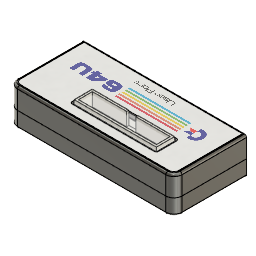
C64U UserPort Case (Autodesk Fusion 360 design; units mm, degrees)
part number: 2026-07-06-14-41-17-070
part number: 2026-07-06-14-41-58-106
part number: 2026-07-06-16-35-42-288
part number: 2026-07-06-17-32-42-446
part number: 2026-07-06-18-13-47-338
Autodesk Fusion 360 part; units mm, degrees
note: some values were not read from the file. Chosen so that the rebuilt part matches the saved one: which bodies a step acts on; the layout of a text. Set by a fixed rule: which sketch regions a step uses.
sketch "Sketch1" plane through (0, 0, 0) normal (0, 0, 1) x (1, 0, 0) in component "PCB"
  line L0 (49.1, 33.3) -> (2, 33.3)
  line L1 (0, 31.3) -> (0, 2)
  arc A0 (2, 33.3) -> (0, 31.3) centre (2, 31.3) ccw
  arc A1 (51.1, 31.3) -> (49.1, 33.3) centre (49.1, 31.3) ccw
  arc A2 (0, 2) -> (2, 0) centre (2, 2) ccw
  arc A3 (49.1, 0) -> (51.1, 2) centre (49.1, 2) ccw
  arc A4 (7.5, 0) -> (4.5, 0) centre (6, 0) ccw
  line L2 (2, 0) -> (4.5, 0)
  line L3 (7.5, 0) -> (49.1, 0)
  arc A5 (51.1, 20) -> (51.1, 17) centre (51.1, 18.5) ccw
  line L4 (51.1, 2) -> (51.1, 17)
  line L5 (51.1, 20) -> (51.1, 31.3)
  line L6 (9.9, 4.5) -> (50.4, 4.5)
  line L7 (50.4, 4.5) -> (50.4, 13.5)
  line L8 (50.4, 13.5) -> (9.9, 13.5)
  line L9 (9.9, 13.5) -> (9.9, 4.5)
  line L10 (11, 5.6) -> (49.3, 5.6)
  line L11 (49.3, 5.6) -> (49.3, 12.4)
  line L12 (49.3, 12.4) -> (11, 12.4)
  line L13 (11, 12.4) -> (11, 5.6)
  line L14 (30.15, 13.5) -> (30.15, 4.5) construction
  line L15 (32.4, 12.4) -> (32.4, 13.5)
  line L16 (27.9, 13.5) -> (27.9, 12.4)
  line L17 (14.55, 21.8) -> (36.55, 21.8)
  line L18 (36.55, 21.8) -> (36.55, 19.8)
  line L19 (36.55, 19.8) -> (14.55, 19.8)
  line L20 (14.55, 19.8) -> (14.55, 21.8)
  line L21 (25.55, 33.3) -> (25.55, 0) construction
  dimension "d3" = 2
  dimension "d4" = 2
  dimension "d5" = 2
  dimension "d6" = 2
  dimension "d7" = 33.3
  dimension "d8" = 51.1
  dimension "d9" = 3
  dimension "d10" = 6
  dimension "d11" = 3
  dimension "d12" = 18.5
  dimension "d13" = 40.5
  dimension "d14" = 9
  dimension "d15" = 0.7
  dimension "d16" = 4.5
  dimension "d17" = -1.1
  dimension "d18" = 4.5
  dimension "d19" = 22
  dimension "d20" = 2
  dimension "d21" = 11.5
  constraint horizontal L2
  constraint vertical L4
  constraint horizontal L0
  constraint vertical L1
  constraint tangent L0 A0
  constraint tangent L1 A0
  constraint tangent A1 L5
  constraint tangent L0 A1
  constraint tangent A2 L2
  constraint tangent L1 A2
  constraint tangent A3 L3
  constraint tangent A3 L4
  constraint coincident A4.centre L2
  constraint collinear L2 L3
  constraint coincident A5.centre L4
  constraint collinear L4 L5
  constraint horizontal L6
  constraint vertical L7
  constraint horizontal L8
  constraint vertical L9
  constraint midpoint L8 L14.start
  constraint midpoint L6 L14.end
  constraint coincident L12 L15.start
  constraint coincident L8 L15.end
  constraint perpendicular L8 L15
  constraint coincident L8 L16.start
  constraint coincident L12 L16.end
  constraint perpendicular L12 L16
  constraint symmetric L14 L15 L16
  constraint horizontal L17
  constraint vertical L18
  constraint horizontal L19
  constraint vertical L20
  constraint midpoint L0 L21.start
  constraint coincident L3 L21.end
  constraint perpendicular L3 L21
  constraint symmetric L18 L20 L21
  measures "d3" radius of A0
  measures "d4" radius of A1
  measures "d5" radius of A2
  measures "d6" radius of A3
  measures "d7" distance of L0 L2
  measures "d8" distance of L1 L4
  measures "d9" diameter of A4
  measures "d10" distance of L1 A4.centre
  measures "d11" diameter of A5
  measures "d12" distance of L3 A5.centre
  measures "d13" distance of L7 L9
  measures "d14" distance of L6.end L7.end
  measures "d15" distance of L4 L7
  measures "d16" distance of L3 L6
  measures "d18" distance of L15 L16
  measures "d19" distance of L18 L20
  measures "d20" distance of L17 L19
  measures "d21" distance of L0 L17
extrude "Extrude1" add sketch "Sketch1" against normal blind 1.6 contours L0 L1 A0 A1 A2 A3 A4 L2 L3 A5 L4 L5 | L6 L7 L8 L9 L10 L11 L12 L13 L15 L16 | L8 L12 L15 L16 | L10 L11 L12 L13 | L17 L18 L19 L20 makes body 1 in component "PCB"
extrude "Extrude2" add sketch "Sketch1" along normal blind 9.5 contours L6 L7 L8 L9 L10 L11 L12 L13 L15 L16 bodies 1 in component "PCB"
extrude "Extrude3" add sketch "Sketch1" along normal blind 3 contours L8 L12 L15 L16 | L10 L11 L12 L13 bodies 1 in component "PCB"
ref_plane "WorkPlane1" through (25.55, 16.65, -7.9) normal (0, 0, 1) x (1, 0, 0) in component "bottom_shell"
sketch "Sketch1 (2)" plane through (0, 0, -7.9) normal (0, 0, 1) x (1, 0, 0) in component "bottom_shell"
  line L0 (49.1, 33.3) -> (2, 33.3) construction
  arc A0 (2, 33.3) -> (0, 31.3) centre (2, 31.3) ccw construction
  line L1 (0, 31.3) -> (0, 2) construction
  arc A1 (0, 2) -> (2, 0) centre (2, 2) ccw construction
  line L2 (2, 0) -> (4.5, 0) construction
  arc A2 (7.5, 0) -> (4.5, 0) centre (6, 0) ccw construction
  line L3 (7.5, 0) -> (49.1, 0) construction
  arc A3 (49.1, 0) -> (51.1, 2) centre (49.1, 2) ccw construction
  line L4 (51.1, 2) -> (51.1, 17) construction
  arc A4 (51.1, 20) -> (51.1, 17) centre (51.1, 18.5) ccw construction
  line L5 (51.1, 20) -> (51.1, 31.3) construction
  arc A5 (51.1, 31.3) -> (49.1, 33.3) centre (49.1, 31.3) ccw construction
  line L6 (25.55, 33.3) -> (25.55, 0) construction
  line L7 (50.4, 13.5) -> (9.9, 13.5) construction
  line L8 (9.9, 13.5) -> (9.9, 4.5) construction
  line L9 (9.9, 4.5) -> (50.4, 4.5) construction
  line L10 (50.4, 4.5) -> (50.4, 13.5) construction
  line L11 (14.55, 21.8) -> (36.55, 21.8) construction
  line L12 (36.55, 19.8) -> (14.55, 19.8) construction
  circle A6 centre (-4.5, 17.8) radius 4
  circle A7 centre (-4.5, 3.5) radius 4
  line L13 (-14.95, 33.3) -> (66.05, 33.3)
  line L14 (66.05, 33.3) -> (66.05, 1.5)
  line L15 (62.05, -2.5) -> (-10.95, -2.5)
  line L16 (-14.95, 1.5) -> (-14.95, 33.3)
  line L17 (-12.95, 33.3) -> (-12.95, 1.5)
  line L18 (-10.95, -0.5) -> (62.05, -0.5)
  line L19 (64.05, 1.5) -> (64.05, 33.3)
  arc A8 (-12.95, 1.5) -> (-10.95, -0.5) centre (-10.95, 1.5) ccw
  arc A9 (62.05, -0.5) -> (64.05, 1.5) centre (62.05, 1.5) ccw
  arc A10 (-14.95, 1.5) -> (-10.95, -2.5) centre (-10.95, 1.5) ccw
  arc A11 (62.05, -2.5) -> (66.05, 1.5) centre (62.05, 1.5) ccw
  line L20 (4.8, 0) -> (4.8, -0.5)
  line L21 (7.2, 0) -> (7.2, -0.5)
  arc A12 (7.2, -0.0006) -> (4.8, 0) centre (6, 0) ccw
  line L22 (6, 0) -> (6, -0.5) construction
  line L23 (3.5, -0.5) -> (8.5, -0.5)
  line L24 (8.5, -0.5) -> (8.5, 2.5)
  line L25 (8.5, 2.5) -> (3.5, 2.5)
  line L26 (3.5, 2.5) -> (3.5, -0.5)
  line L27 (-12.95, 7.5) -> (2.5, 7.5)
  line L28 (2.5, 7.5) -> (2.5, -0.5)
  line L29 (-0.3, 7.5) -> (-0.3, -0.5)
  line L30 (-12.95, 21.8) -> (2.5, 21.8)
  line L31 (2.5, 21.8) -> (2.5, 13.8)
  line L32 (2.5, 13.8) -> (-12.95, 13.8)
  line L33 (-0.3, 21.8) -> (-0.3, 13.8)
  circle A13 centre (-4.5, 17.8) radius 3
  circle A14 centre (-4.5, 3.5) radius 3
  line L34 (64.05, 21.8) -> (48.6, 21.8)
  circle A15 centre (55.6, 17.8) radius 4
  circle A16 centre (55.6, 17.8) radius 3
  line L35 (48.6, 13.8) -> (64.05, 13.8)
  line L36 (51.4, 21.8) -> (51.4, 13.8)
  line L37 (48.6, 21.8) -> (48.6, 13.8)
  line L38 (64.05, 7.5) -> (48.6, 7.5)
  circle A17 centre (55.6, 3.5) radius 4
  circle A18 centre (55.6, 3.5) radius 3
  line L39 (51.4, 7.5) -> (51.4, -0.5)
  line L40 (48.6, 7.5) -> (48.6, -0.5)
  circle A19 centre (-4.5, 17.8) radius 1.75
  circle A20 centre (-4.5, 3.5) radius 1.75
  circle A21 centre (55.6, 17.8) radius 1.75
  circle A22 centre (55.6, 3.5) radius 1.75
  line L41 (2.5, 21.8) -> (48.6, 21.8)
  line L42 (2.5, 19.8) -> (48.6, 19.8)
  line L43 (64.85, 32.1) -> (64.85, 1.5)
  arc A23 (62.05, -1.3) -> (64.85, 1.5) centre (62.05, 1.5) ccw
  line L44 (62.05, -1.3) -> (-10.95, -1.3)
  arc A24 (-13.75, 1.5) -> (-10.95, -1.3) centre (-10.95, 1.5) ccw
  line L45 (-13.75, 1.5) -> (-13.75, 32.1)
  line L46 (-13.75, 32.1) -> (-13.75, 33.3)
  line L47 (64.85, 32.1) -> (64.85, 33.3)
  line L48 (51.1, 20) -> (51.1, 17) construction
  line L49 (51.4, 19.7) -> (51.1, 19.7)
  arc A25 (51.1, 19.7) -> (51.1, 17.3) centre (51.1, 18.5) ccw
  line L50 (51.1, 18.5) -> (50.5645, 18.5) construction
  line L51 (51.4, 17.3) -> (51.1, 17.3)
  point P0 (4.5, 0)
  dimension "d34" = 8
  dimension "d35" = 8
  dimension "d37" = 4.5
  dimension "d39" = 4.5
  dimension "d41" = 4
  dimension "d42" = 2.5
  dimension "d43" = 81
  dimension "d44" = 2
  dimension "d45" = 2
  dimension "d46" = 2
  dimension "d47" = 2
  dimension "d48" = 4
  dimension "d49" = 4
  dimension "d50" = 0.3
  dimension "d51" = 0.3
  dimension "d52" = 5
  dimension "d53" = 3
  dimension "d54" = 2.5
  dimension "d55" = 0.3
  dimension "d56" = 6
  dimension "d57" = 6
  dimension "d58" = 3.5
  dimension "d59" = 3.5
  dimension "d60" = 2
  dimension "d61" = 1.2
  dimension "d63" = 0.3
  constraint horizontal L13
  constraint vertical L14
  constraint horizontal L15
  constraint vertical L16
  constraint collinear L0 L13
  constraint symmetric L6 L14 L16
  constraint coincident L13 L17.start
  constraint perpendicular L13 L17
  constraint perpendicular L14 L18
  constraint coincident L13 L19.end
  constraint perpendicular L13 L19
  constraint symmetric L6 L17 L19
  constraint tangent L17 A8
  constraint tangent L18 A8
  constraint tangent L18 A9
  constraint tangent L19 A9
  constraint tangent L15 A10
  constraint tangent L16 A10
  constraint tangent L14 A11
  constraint tangent L15 A11
  constraint concentric A2 A12
  constraint coincident L18 L20.end
  constraint perpendicular L18 L20
  constraint coincident L21.start A12
  constraint coincident L18 L21.end
  constraint perpendicular L18 L21
  constraint coincident L21 A12.start
  constraint coincident A2.centre A12.centre
  constraint coincident L18 L22.end
  constraint perpendicular L18 L22
  constraint horizontal L23
  constraint vertical L24
  constraint horizontal L25
  constraint vertical L26
  constraint coincident L18 L23.start
  constraint symmetric L22 L24 L26
  constraint coincident L17 L27.start
  constraint perpendicular L1 L27
  constraint coincident L18 L28.end
  constraint perpendicular L18 L28
  constraint tangent A7 L27
  constraint coincident L27 L29.start
  constraint coincident L18 L29.end
  constraint perpendicular L18 L29
  constraint coincident L17 L30.start
  constraint perpendicular L1 L30
  constraint perpendicular L30 L31
  constraint coincident L17 L32.end
  constraint perpendicular L17 L32
  constraint collinear L28 L31
  constraint tangent A6 L30
  constraint tangent A6 L32
  constraint coincident L30 L33.start
  constraint coincident L32 L33.end
  constraint perpendicular L32 L33
  constraint collinear L29 L33
  constraint concentric A6 A13
  constraint tangent A7 L18
  constraint concentric A7 A14
  constraint symmetric L6 A6 A15
  constraint symmetric L6 A7 A17
  constraint symmetric L6 L27.start L38.start
  constraint symmetric L6 L27.end L38.end
  constraint symmetric L6 L28.end L40.end
  constraint symmetric L6 L29.start L39.start
  constraint symmetric L6 L29.end L39.end
  constraint symmetric L6 L30.start L34.start
  constraint symmetric L6 L30.end L34.end
  constraint symmetric L6 L31.end L35.start
  constraint symmetric L6 L32.end L35.end
  constraint symmetric L6 L33.start L36.start
  constraint symmetric L6 L33.end L36.end
  constraint symmetric L6 A13 A16
  constraint symmetric L6 A14 A18
  constraint concentric A13 A19
  constraint concentric A14 A20
  constraint symmetric L6 A19 A21
  constraint symmetric L6 A20 A22
  constraint coincident L31 L42.start
  constraint coincident L37 L42.end
  constraint perpendicular L37 L42
  constraint coincident L13 L46.end
  constraint perpendicular L13 L46
  constraint perpendicular L13 L47
  constraint concentric A4 A25
  constraint coincident A4.start L5.start
  constraint coincident L4.end A4.end
  constraint coincident L36 L49.start
  constraint perpendicular L48 L49
  constraint tangent L49 A25
  constraint coincident L48 A25.end
  constraint coincident A4.centre A25.centre
  constraint perpendicular L48 L50
  constraint symmetric L49.start L50 L51.start
  constraint symmetric L49.end L50 A25.end
  measures "d34" diameter of A6
  measures "d35" diameter of A7
  measures "d37" distance of L1 A6.centre
  measures "d39" distance of L1 A7.centre
  measures "d41" distance of L11 A6.centre
  measures "d42" distance of L3 L15
  measures "d43" distance of L13.start L13.end
  measures "d44" distance of L16 L17
  measures "d45" distance of L15 L18
  measures "d46" radius of A8
  measures "d47" radius of A9
  measures "d48" radius of A10
  measures "d49" radius of A11
  measures "d50" distance of A2 A12
  measures "d51" distance of L20 P0
  measures "d52" distance of L24 L26
  measures "d53" distance of L18 L25
  measures "d54" distance of L1 L28
  measures "d55" distance of L1 L29
  measures "d56" diameter of A13
  measures "d57" diameter of A14
  measures "d58" diameter of A19
  measures "d59" diameter of A20
  measures "d60" distance of L41 L42
  measures "d63" distance of A4 A25
extrude "Extrude3'" add sketch "Sketch1 (2)" against normal blind 2 separate body contours A6 | A6 L30 L32 L33 | A6 L17 L30 L32 | L13 L17 L19 L30 L34 L41 | L17 L18 L19 L24 L25 L26 L27 L28 L31 L32 L35 L37 L38 L40 L42 | L13 L17 L18 L19 A8 A9 L23 L43 A23 L44 A24 L45 L46 L47 | L30 L31 L32 L33 | L31 L37 L41 L42 | A7 L17 L18 A8 L27 | L13 L14 L15 L16 A10 A11 L43 A23 L44 A24 L45 L46 L47 | L34 L35 L36 L37 L49 A25 L51 | A7 L18 L27 L29 | A7 | L19 L34 A15 L35 | L34 A15 L35 L36 | L18 L27 L28 L29 | A15 | L36 L49 A25 L51 | L18 L19 A9 L38 A17 | L18 L38 A17 L39 | A17 | L18 L20 L21 A12 L23 L24 L25 L26 | L18 L38 L39 L40 | L18 L20 L21 A12 L23 makes body 2 in component "bottom_shell"
extrude "Extrude1'" add sketch "Sketch1 (2)" along normal blind 6.3 separate body contours L30 L31 L32 L33 | L31 L37 L41 L42 | L34 L35 L36 L37 L49 A25 L51 | L18 L27 L28 L29 | L18 L20 L21 A12 L23 L24 L25 L26 | L18 L38 L39 L40 makes body 3 at (5.1667, 2.5, -3.7) makes body 4 at (51.4, 4.8333, -5.8) makes body 5 at (2.5, 4.8333, -5.8) makes body 6 at (34.1667, 21.8, -3.7) in component "bottom_shell"
extrude "Extrude2'" add sketch "Sketch1 (2)" along normal blind 7.9 separate body contours A6 | A6 L30 L32 L33 | A6 L17 L30 L32 | L13 L17 L18 L19 A8 A9 L23 L43 A23 L44 A24 L45 L46 L47 | A7 L17 L18 A8 L27 | A7 L18 L27 L29 | A7 | L19 L34 A15 L35 | L34 A15 L35 L36 | A15 | L36 L49 A25 L51 | L18 L19 A9 L38 A17 | L18 L38 A17 L39 | A17 | L18 L20 L21 A12 L23 makes body 7 in component "bottom_shell"
extrude "Extrude4" add sketch "Sketch1 (2)" along normal blind 4.6 from surface at 3.3 contours A13 | A14 | A16 | A18 bodies 7 in component "bottom_shell"
extrude "Extrude5" add sketch "Sketch1 (2)" along normal blind 5.9 contours L13 L14 L15 L16 A10 A11 L43 A23 L44 A24 L45 L46 L47 bodies 7 2 in component "bottom_shell"
fillet "Fillet1" radius 1 12 edges at (8.5, 2.5, -4.75) (3.5, 2.5, -4.75) (48.6, 7.5, -4.75) (2.5, 7.5, -4.75) (2.5, 13.8, -4.75) (48.6, 13.8, -4.75) (64.05, 21.8, -3.95) (-12.95, 21.8, -3.95) (64.05, 7.5, -3.95) (64.05, 13.8, -3.95) (-12.95, 7.5, -3.95) (-12.95, 13.8, -3.95) on bodies 3 4 5 6 7 in component "bottom_shell"
fillet "Fillet2" radius 1 5 edges at (66.05, 17.4, -9.9) (64.8784, -1.3284, -9.9) (25.55, -2.5, -9.9) (-13.7784, -1.3284, -9.9) (-14.95, 17.4, -9.9) on bodies 7 in component "bottom_shell"
ref_plane "WorkPlane1" through (25.55, 27.55, 6.1) normal (0, 0, 1) x (1, 0, 0) in component "top_shell"
sketch "Sketch1 (3)" plane through (0, 0, 6.1) normal (0, 0, 1) x (1, 0, 0) in component "top_shell"
  arc A0 (62.05, -2.5) -> (66.05, 1.5) centre (62.05, 1.5) ccw
  line L0 (62.05, -2.5) -> (-10.95, -2.5)
  arc A1 (-14.95, 1.5) -> (-10.95, -2.5) centre (-10.95, 1.5) ccw
  line L1 (-14.95, 1.5) -> (-14.95, 33.3)
  line L2 (-14.95, 33.3) -> (66.05, 33.3)
  line L3 (64.05, 1.5) -> (64.05, 33.3)
  line L4 (66.05, 33.3) -> (66.05, 1.5)
  arc A2 (62.05, -0.5) -> (64.05, 1.5) centre (62.05, 1.5) ccw
  line L5 (-10.95, -0.5) -> (62.05, -0.5)
  arc A3 (-12.95, 1.5) -> (-10.95, -0.5) centre (-10.95, 1.5) ccw
  line L6 (-12.95, 33.3) -> (-12.95, 1.5)
  line L7 (64.05, 21.8) -> (48.6, 21.8)
  line L8 (2.5, 19.8) -> (48.6, 19.8) construction
  line L9 (2.5, 21.8) -> (48.6, 21.8)
  line L10 (2.5, 21.8) -> (2.5, 13.8) construction
  line L11 (2.5, 13.8) -> (-12.95, 13.8) construction
  line L12 (-12.95, 21.8) -> (2.5, 21.8)
  line L13 (-12.95, 7.5) -> (2.5, 7.5) construction
  line L14 (2.5, 7.5) -> (2.5, -0.5) construction
  line L15 (8.5, 2.5) -> (3.5, 2.5)
  line L16 (3.5, 2.5) -> (3.5, -0.5)
  line L17 (8.5, -0.5) -> (8.5, 2.5)
  line L18 (64.05, 7.5) -> (48.6, 7.5) construction
  line L19 (48.6, 7.5) -> (48.6, -0.5) construction
  circle A4 centre (-4.5, 3.5) radius 1.75 construction
  circle A5 centre (-4.5, 17.8) radius 1.75 construction
  circle A6 centre (55.6, 17.8) radius 1.75 construction
  circle A7 centre (55.6, 3.5) radius 1.75 construction
  line L20 (51.1, 2) -> (51.1, 17) construction
  line L21 (9.9, 4.5) -> (50.4, 4.5) construction
  line L22 (50.4, 4.5) -> (50.4, 13.5) construction
  line L23 (50.4, 13.5) -> (9.9, 13.5) construction
  line L24 (9.9, 13.5) -> (9.9, 4.5) construction
  line L25 (0, 31.3) -> (0, 2) construction
  circle A8 centre (55.6, 3.5) radius 1.25
  circle A9 centre (55.6, 17.8) radius 1.25
  circle A10 centre (-4.5, 3.5) radius 1.25
  line L26 (0.5, -0.5) -> (0.5, 7.5)
  line L27 (0.5, 7.5) -> (-12.95, 7.5)
  line L28 (0.5, 13.8) -> (0.5, 21.8)
  line L29 (0.5, 13.8) -> (-12.95, 13.8)
  line L30 (50.9, 14) -> (9.4, 14)
  line L31 (9.4, 14) -> (9.4, 4)
  line L32 (9.4, 4) -> (50.9, 4)
  line L33 (50.9, 4) -> (50.9, 14)
  line L34 (50.9, 14) -> (64.05, 14)
  line L35 (48.6, 21.8) -> (48.6, 14)
  line L36 (64.05, 7.5) -> (50.9, 7.5)
  line L37 (48.6, 4) -> (48.6, -0.5)
  arc A11 (62.05, -1.7) -> (65.25, 1.5) centre (62.05, 1.5) ccw
  line L38 (65.25, 33.3) -> (65.25, 1.5)
  line L39 (-14.15, 1.5) -> (-14.15, 33.3)
  arc A12 (-14.15, 1.5) -> (-10.95, -1.7) centre (-10.95, 1.5) ccw
  line L40 (62.05, -1.7) -> (-10.95, -1.7)
  line L41 (65.25, 33.3) -> (65.25, 33.3)
  line L42 (-14.15, 33.3) -> (-14.15, 33.3)
  line L43 (48.6, 19.8) -> (0.5, 19.8)
  line L44 (42.1, 19.8) -> (42.1, 21.8)
  line L45 (15, 19.8) -> (15, 21.8)
  circle A13 centre (-4.5, 17.8) radius 1.25
  dimension "d81" = 2.5
  dimension "d82" = 2.5
  dimension "d83" = 2.5
  dimension "d84" = 0.5
  dimension "d85" = 0.5
  dimension "d86" = 0.8
  dimension "d87" = 15
  dimension "d88" = 9
  dimension "d113" = 2.5
  constraint concentric A7 A8
  constraint concentric A6 A9
  constraint concentric A4 A10
  constraint coincident L5 L26.start
  constraint coincident L13 L26.end
  constraint coincident L13.start L27.end
  constraint perpendicular L5 L26
  constraint coincident L11 L28.start
  constraint coincident L12 L28.end
  constraint perpendicular L12 L28
  constraint collinear L26 L28
  constraint coincident L11.end L29.end
  constraint coincident L3 L34.end
  constraint perpendicular L3 L34
  constraint coincident L7.end L9.end
  constraint coincident L30 L35.end
  constraint perpendicular L30 L35
  constraint coincident L18.start L36.start
  constraint coincident L18 L36.end
  constraint coincident L33 L36.end
  constraint coincident L19 L37.start
  constraint coincident L32 L37.start
  constraint coincident L19.end L37.end
  constraint coincident L2 L38.start
  constraint perpendicular L2 L41
  constraint coincident L2 L39.end
  constraint perpendicular L2 L42
  constraint coincident L8.end L43.start
  constraint coincident L28 L43.end
  constraint perpendicular L28 L43
  constraint coincident L43 L44.start
  constraint coincident L9 L44.end
  constraint perpendicular L9 L44
  constraint coincident L8 L45.start
  constraint coincident L9 L45.end
  constraint perpendicular L9 L45
  constraint concentric A5 A13
  measures "d81" diameter of A8
  measures "d82" diameter of A9
  measures "d83" diameter of A10
  measures "d84" distance of L25 L26
  measures "d87" distance of L25 L45
  measures "d88" distance of L20 L44
  measures "d113" diameter of A13
extrude "Extrude1''" add sketch "Sketch1 (3)" along normal blind 2 separate body contours A0 L0 A1 L1 L2 L4 A11 L38 L39 A12 L40 | L2 L3 A2 L5 A3 L6 A11 L38 L39 A12 L40 | L2 L3 L6 L7 L9 L12 | L3 L7 L30 L34 L35 | L6 L12 L28 L29 | L3 L33 L34 L36 | L9 L35 L43 L44 | L5 L6 L15 L16 L17 L26 L27 L28 L29 L30 L31 L32 L35 L37 L43 | L9 L12 L28 L43 L45 | L3 A2 L5 L32 L33 L36 L37 | L9 L43 L44 L45 | L5 A3 L6 L26 L27 | L5 L15 L16 L17 | A8 | A9 | A10 | A13 makes body 8 in component "top_shell"
extrude "Extrude2''" add sketch "Sketch1 (3)" against normal blind 6.1 contours L2 L3 A2 L5 A3 L6 A11 L38 L39 A12 L40 | L3 L7 L30 L34 L35 | L6 L12 L28 L29 | L3 A2 L5 L32 L33 L36 L37 | L9 L43 L44 L45 | L5 A3 L6 L26 L27 | L5 L15 L16 L17 bodies 8 in component "top_shell"
extrude "Extrude3''" add sketch "Sketch1 (3)" against normal blind 4.6 contours L9 L35 L43 L44 | L9 L12 L28 L43 L45 bodies 8 in component "top_shell"
extrude "Extrude4'" add sketch "Sketch1 (3)" against normal blind 8.1 contours A0 L0 A1 L1 L2 L4 A11 L38 L39 A12 L40 bodies 8 in component "top_shell"
fillet "Fillet1'" radius 1 15 edges at (-12.95, 7.5, 3.05) (0.5, 7.5, 3.05) (0.5, -0.5, 3.05) (3.5, -0.5, 3.05) (3.5, 2.5, 3.05) (8.5, 2.5, 3.05) (8.5, -0.5, 3.05) (48.6, -0.5, 3.05) (48.6, 4, 3.05) (50.9, 7.5, 3.05) (64.05, 7.5, 3.05) (64.05, 14, 3.05) (48.6, 14, 3.05) (64.05, 21.8, 3.05) (-12.95, 21.8, 3.05) on bodies 8 in component "top_shell"
fillet "Fillet2'" radius 1 3 edges at (0.5, 13.8, 3.05) (0.5, 19.8, 3.8) (-12.95, 13.8, 3.05) on bodies 8 in component "top_shell"
fillet "Fillet3" radius 1 1 edges at (48.6, 19.8, 3.8) on bodies 8 in component "top_shell"
fillet "Fillet4" radius 0.5 4 edges at (42.1, 19.8, 0.75) (42.1, 21.8, 0.75) (15, 21.8, 0.75) (15, 19.8, 0.75) on bodies 8 in component "top_shell"
fillet "Fillet5" radius 0.5 1 edges at (0.5, 21.8, 0.75) on bodies 8 in component "top_shell"
fillet "Fillet6" radius 0.5 1 edges at (48.6, 21.8, 0.75) on bodies 8 in component "top_shell"
fillet "Fillet7" radius 1 5 edges at (-14.95, 17.4, 8.1) (-13.7784, -1.3284, 8.1) (25.55, -2.5, 8.1) (64.8784, -1.3284, 8.1) (66.05, 17.4, 8.1) on bodies 8 in component "top_shell"
fillet "Fillet8" radius 0.5 4 edges at (9.4, 14, 7.1) (9.4, 4, 7.1) (50.9, 4, 4.05) (50.9, 14, 7.1) on bodies 8 in component "top_shell"
sketch "Sketch1 (4)" plane through (0, 0, 8.1) normal (0, 0, 1) x (-1, 0, 0) in component "label"
  line L0 (13.95, -33.3) -> (13.95, -1.5) construction
  arc A0 (13.95, -1.5) -> (10.95, 1.5) centre (10.95, -1.5) ccw construction
  line L1 (10.95, 1.5) -> (-62.05, 1.5) construction
  arc A1 (-62.05, 1.5) -> (-65.05, -1.5) centre (-62.05, -1.5) ccw construction
  line L2 (-65.05, -1.5) -> (-65.05, -33.3) construction
  line L3 (-65.05, -33.3) -> (13.95, -33.3) construction
  line L4 (-50.9, -13.5) -> (-50.9, -4.5) construction
  arc A2 (-50.4, -4) -> (-50.9, -4.5) centre (-50.4, -4.5) ccw construction
  line L5 (-50.4, -4) -> (-9.9, -4) construction
  arc A3 (-9.4, -4.5) -> (-9.9, -4) centre (-9.9, -4.5) ccw construction
  line L6 (-9.4, -4.5) -> (-9.4, -13.5) construction
  arc A4 (-9.9, -14) -> (-9.4, -13.5) centre (-9.9, -13.5) ccw construction
  line L7 (-9.9, -14) -> (-50.4, -14) construction
  arc A5 (-50.9, -13.5) -> (-50.4, -14) centre (-50.4, -13.5) ccw construction
  arc A6 (-62.05, 1.5) -> (-65.05, -1.5) centre (-62.05, -1.5) ccw construction
  line L8 (-62.05, 1.5) -> (10.95, 1.5) construction
  line L9 (-65.05, -33.3) -> (-65.05, -1.5) construction
  line L10 (-65.05, -33.3) -> (13.95, -33.3) construction
  line L11 (13.95, -1.5) -> (13.95, -33.3) construction
  arc A7 (13.95, -1.5) -> (10.95, 1.5) centre (10.95, -1.5) ccw construction
  line L12 (-64.55, -1.5) -> (-64.55, -32.8)
  line L13 (-64.55, -32.8) -> (13.45, -32.8)
  line L14 (13.45, -32.8) -> (13.45, -1.5)
  arc A8 (13.45, -1.5) -> (10.95, 1) centre (10.95, -1.5) ccw
  line L15 (10.95, 1) -> (-62.05, 1)
  arc A9 (-62.05, 1) -> (-64.55, -1.5) centre (-62.05, -1.5) ccw
  arc A10 (-8.9, -4.5) -> (-9.9, -3.5) centre (-9.9, -4.5) ccw
  line L16 (-50.4, -3.5) -> (-9.9, -3.5)
  arc A11 (-50.4, -3.5) -> (-51.4, -4.5) centre (-50.4, -4.5) ccw
  line L17 (-51.4, -13.5) -> (-51.4, -4.5)
  arc A12 (-51.4, -13.5) -> (-50.4, -14.5) centre (-50.4, -13.5) ccw
  line L18 (-9.9, -14.5) -> (-50.4, -14.5)
  arc A13 (-9.9, -14.5) -> (-8.9, -13.5) centre (-9.9, -13.5) ccw
  line L19 (-8.9, -4.5) -> (-8.9, -13.5)
  dimension "d114" = -0.5
  dimension "d115" = -0.5
extrude "Extrude1'''" add sketch "Sketch1 (4)" along normal blind 0.1 separate body makes body 9 in component "label"
ref_plane "WorkPlane2" through (25.55, 15.4, -9.9) normal (0, 0, -1) x (-1, 0, 0) in component "bottom_shell"
ref_plane "WorkPlane1" through (25.55, 15.4, -9.9) normal (0, 0, -1) x (-1, 0, 0)
sketch "Sketch1 (5)" plane through (0, 0, -9.9) normal (0, 0, -1) x (-1, 0, 0)
  line L0 (-4.7329, 31.3197) -> (-47.7329, 31.3197) construction
  line L1 (-47.7329, 31.3197) -> (-47.7329, 22.3197) construction
  line L2 (-47.7329, 22.3197) -> (-4.7329, 22.3197) construction
  line L3 (-4.7329, 22.3197) -> (-4.7329, 31.3197) construction
  dimension "d122" = 7
  text T0 "BOTTOM" font "Arial" height 7 align left top in box 43 x 9 at (-4.7329, 31.3197) x (-1, 0) y (0, -1) spacing 1 kerned
extrude "Extrude6" cut sketch "Sketch1 (5)" against normal blind 0.4 text T0 bodies 7 in component "bottom_shell"
component "PCB" placed x (1, 0, 0) y (0, 1, 0) z (0, 0, 1) at (0, 0, 0)
component "bottom_shell" placed x (1, 0, 0) y (0, 1, 0) z (0, 0, 1) at (0, 0, 0)
component "top_shell" placed x (1, 0, 0) y (0, 1, 0) z (0, 0, 1) at (0, 0, 0)
component "label" placed x (1, 0, 0) y (0, 1, 0) z (0, 0, 1) at (0, 0, 0)
equation "pcb = 1.6 mm"
equation "below = 6.3 mm"
equation "cutoutx = 72 mm"
equation "cutouty = 14 mm"
equation "wall = 2 mm"
equation "d33 = -pcb - below"
equation "d35 = d34"
equation "d37 = d34 / 2 + 0.5 mm"
equation "d39 = d37"
equation "d41 = d34 / 2"
equation "d42 = wall + 0.5 mm"
equation "d43 = 77 mm + 2 * wall"
equation "d44 = wall"
equation "d45 = wall"
equation "d48 = 2 mm + wall"
equation "d49 = d48"
equation "d51 = d50"
equation "d57 = d56"
equation "d60 = wall"
equation "d61 = 0.6 * wall"
equation "overlap = 2 mm"
equation "d63 = d50"
equation "d64 = below"
equation "d66 = below + pcb"
equation "d68 = -wall"
equation "d70 = below - 3 mm"
equation "d71 = 3 mm + pcb"
equation "d73 = below + pcb - overlap"
equation "d79 = cutouty"
equation "above = cutouty - below - pcb"
equation "d82 = d81"
equation "d83 = d81"
equation "d86 = 0.4 * wall"
equation "d89 = wall"
equation "d91 = -above"
equation "d93 = -above + 1.5 mm"
equation "d95 = -above - overlap"
equation "d113 = d83"
equation "d123 = 'BOTTOM'"
